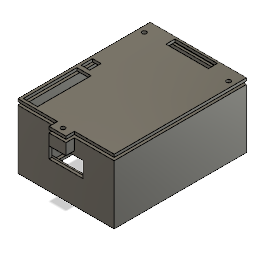
gpsAntenna v12 (Autodesk Fusion 360 design; units mm, degrees)
Autodesk Fusion 360 part; units mm, degrees
sketch "Sketch1" plane through (0, 0, 0) normal (0, 1, 0) x (1, 0, 0)
  line L0 (0, 0) -> (28.2, 0)
  line L1 (28.2, 0) -> (28.2, -28.2)
  line L2 (28.2, -28.2) -> (0, -28.2)
  line L3 (0, -28.2) -> (0, 0)
  line L4 (29.7, -29.7) -> (-1.5, -29.7)
  line L5 (-1.5, -29.7) -> (-1.5, 1.5)
  line L6 (-1.5, 1.5) -> (29.7, 1.5)
  line L7 (29.7, 1.5) -> (29.7, -29.7)
  line L8 (26.7, -1.5) -> (26.3464, -1.8536) construction
  line L9 (26.3464, -1.8536) -> (26.7, -2.2071) construction
  line L10 (26.7, -2.2071) -> (25.9929, -1.5)
  line L11 (26.7, -1.5) -> (27.0536, -1.1464) construction
  circle A0 centre (27.0536, -1.1464) radius 0.75
  line L12 (26.7, -26.7) -> (1.5, -1.5) construction
  line L13 (1.5, -26.7) -> (26.7, -1.5) construction
  circle A1 centre (1.1464, -1.1464) radius 0.75
  circle A2 centre (1.1464, -27.0536) radius 0.75
  circle A3 centre (27.0536, -27.0536) radius 0.75
  line L14 (27.2, -27.2) -> (1, -27.2)
  line L15 (1, -27.2) -> (1, -1)
  line L16 (1, -1) -> (27.2, -1)
  line L17 (27.2, -1) -> (27.2, -27.2)
  line L18 (27.2, -2.7071) -> (25.4929, -1)
  line L19 (2.7071, -1) -> (1, -2.7071)
  line L20 (1, -25.4929) -> (2.7071, -27.2)
  line L21 (25.4929, -27.2) -> (27.2, -25.4929)
  dimension "d1" = 28.2
  dimension "d2" = 28.2
  dimension "d5" = 1.5
  dimension "d12" = 1.5
  dimension "d15" = 1
  dimension "d17" = 360
  measures "d12" diameter of A0
extrude "Extrude1" add sketch "Sketch1" along normal blind 1 contours L0 L1 L2 L3 | L4 L5 L6 L7 | A3 L14 L17 L21 | A1 L15 L16 L19 | A2 L14 L15 L20 makes body 1
extrude "Extrude2" add sketch "Sketch1" along normal blind 5 contours L4 L5 L6 L7 bodies 1
extrude "Extrude3" add sketch "Sketch1" along normal blind 1 contours L10 A0 L16 L17 L18 bodies 1
extrude "Extrude4" add 1 faces at (-1, 5, 9.4) along direction (0, 1, 0) blind 1 on bodies 1 bodies 1
ref_plane "WorkPlane1" through (14.1, 6, 14.1) normal (0, 1, 0) x (0, 0, 1)
sketch "Sketch2" plane through (14.1, 6, 14.1) normal (0, 1, 0) x (1, 0, 0)
  line L0 (15.6, -15.6) -> (-15.6, -15.6)
  line L1 (15.6, -15.6) -> (15.6, -26) construction
  line L2 (15.6, -18.25) -> (-15.6, -18.25)
  line L3 (-15.6, -18.25) -> (-15.6, 18.25)
  line L4 (-15.6, 18.25) -> (15.6, 18.25)
  line L5 (15.6, 18.25) -> (15.6, -18.25)
  line L6 (15.6, -18.25) -> (-15.6, 18.25) construction
  line L7 (-15.6, -18.25) -> (15.6, 18.25) construction
  line L8 (16.1, -18.75) -> (-16.1, -18.75)
  line L9 (-16.1, -18.75) -> (-16.1, 18.75)
  line L10 (-16.1, 18.75) -> (16.1, 18.75)
  line L11 (16.1, 18.75) -> (16.1, -18.75)
  line L12 (17.1, -19.75) -> (-17.1, -19.75)
  line L13 (-17.1, -19.75) -> (-17.1, 19.75)
  line L14 (-17.1, 19.75) -> (17.1, 19.75)
  line L15 (17.1, 19.75) -> (17.1, -19.75)
  line L16 (-12.8, 25.4) -> (-12.8, -15.6)
  line L17 (-12.8, -15.6) -> (12.8, -15.6)
  line L18 (12.8, -15.6) -> (12.8, 25.4)
  line L19 (17.1, 19.75) -> (-17.1, 19.75)
  line L20 (-17.1, 19.75) -> (-17.1, 27.25)
  line L21 (-17.1, 27.25) -> (17.1, 27.25)
  line L22 (17.1, 27.25) -> (17.1, 19.75)
  line L23 (-12.8, 25.4) -> (12.8, 25.4)
  line L24 (12.8, 25.4) -> (12.8, 26.4)
  line L25 (12.8, 26.4) -> (-12.8, 26.4)
  line L26 (-12.8, 26.4) -> (-12.8, 25.4)
  dimension "d27" = 31.2
  dimension "d28" = 36.5
  dimension "d29" = 0.5
  dimension "d30" = 1.5
  dimension "d33" = 41
  dimension "d34" = 25.6
  dimension "d35" = 7.5
  dimension "d36" = 1
  measures "d29" distance of L2
  measures "d30" distance of L2
extrude "Extrude5" add sketch "Sketch2" against normal blind 6 separate body contours L8 L9 L10 L11 L12 L13 L14 L15 L16 L18 L19 | L14 L16 L18 L19 L20 L21 L22 L24 L25 L26 makes body 2
extrude "Extrude6" add 1 faces at (-1.5667, 6, -10.0333) along direction (0, 1, 0) blind 13 on bodies 2 bodies 2
extrude "Extrude7" add 1 faces at (-1.5, 2, 19.3) along direction (-1, 0, 0) blind 1.5 on bodies 1 bodies 1 2
extrude "Extrude8" add 1 faces at (29.7, 4, 19.3) along direction (1, 0, 0) blind 1.5 on bodies 1 bodies 1
ref_plane "WorkPlane2" through (14.1, 0, 10.35) normal (0, -1, 0) x (-1, 0, 0)
sketch "Sketch3" plane through (14.1, 0, 10.35) normal (0, -1, 0) x (1, 0, 0)
  line L0 (-17.1, -23.5) -> (17.1, -23.5)
  line L1 (17.1, -23.5) -> (17.1, 23.5)
  line L2 (17.1, 23.5) -> (-17.1, 23.5)
  line L3 (-17.1, 23.5) -> (-17.1, -23.5)
  line L4 (-12.8, -22.65) -> (12.8, -22.65)
  line L5 (12.8, -22.65) -> (12.8, -11.85)
  line L6 (12.8, -11.85) -> (-12.8, -11.85)
  line L7 (-12.8, -11.85) -> (-12.8, -22.65)
  line L8 (12.8, -22.65) -> (-12.8, -22.65)
  line L9 (0, -22.65) -> (0, -11.85)
  line L10 (-11.8, -21.65) -> (11.8, -21.65)
  line L11 (11.8, -21.65) -> (11.8, -12.85)
  line L12 (11.8, -12.85) -> (-11.8, -12.85)
  line L13 (-11.8, -12.85) -> (-11.8, -21.65)
  line L14 (-16.1, 19.35) -> (16.1, 19.35)
  line L15 (16.1, 19.35) -> (16.1, -11.85)
  line L16 (16.1, -11.85) -> (-16.1, -11.85)
  line L17 (-16.1, -11.85) -> (-16.1, 19.35)
  line L18 (-11.8, -12.85) -> (-7.8, -12.85)
  line L19 (-7.8, -12.85) -> (-7.8, -16.85)
  line L20 (-7.8, -16.85) -> (-11.8, -16.85)
  line L21 (-11.8, -16.85) -> (-11.8, -12.85)
  line L22 (0, -21.65) -> (11.8, -12.85) construction
  line L23 (5.9, -17.25) -> (5.9, -21.65) construction
  line L24 (5.9, -21.65) -> (5.9, -22.65) construction
  line L25 (5.9, -22.65) -> (5.9, -11.85)
  dimension "d46" = 1
  dimension "d53" = 4
  dimension "d54" = 4
  measures "d46" distance of L4
extrude "Extrude9" add sketch "Sketch3" against normal blind 0.5 contours L0 L1 L2 L3 | L4 L8 L9 L10 L25 | L4 L5 L6 L8 L10 L11 L12 L16 L25 | L9 L10 L12 L13 L19 L20 | L9 L10 L12 L25 | L6 L9 L12 L16 L25 | L10 L11 L12 L25 | L12 L13 L18 L19 L20 L21 bodies 1
extrude "Extrude10" add sketch "Sketch3" against normal blind 1 contours L9 L10 L12 L13 L19 L20 | L12 L13 L18 L19 L20 L21 bodies 1
extrude "Extrude11" add sketch "Sketch3" against normal blind 1 contours L4 L8 L9 L10 L25 | L4 L5 L6 L8 L10 L11 L12 L16 L25 | L9 L10 L12 L25 | L6 L9 L12 L16 L25 | L10 L11 L12 L25 bodies 1
extrude "Extrude12" add sketch "Sketch3" against normal blind 6 contours L12 L13 L18 L19 L20 L21 bodies 1
extrude "Extrude13" add 1 faces at (-1.2333, 19, -10.0333) along direction (0, 1, 0) blind 2 on bodies 1 bodies 1
ref_plane "WorkPlane3" through (14.1, 21, 10.35) normal (0, 1, 0) x (0, 0, 1)
sketch "Sketch4" plane through (14.1, 21, 10.35) normal (0, 1, 0) x (1, 0, 0)
  line L0 (17.1, -23.5) -> (-17.1, -23.5)
  line L1 (-17.1, -23.5) -> (-17.1, 23.5)
  line L2 (-17.1, 23.5) -> (17.1, 23.5)
  line L3 (17.1, 23.5) -> (17.1, -23.5)
  line L4 (-12.8, 15) -> (-17.1, 23.5)
  circle A0 centre (-14.95, 19.25) radius 0.75
  line L5 (16.1, 15) -> (16.1, -22.5)
  line L6 (0, 0) -> (0, -7)
  circle A1 centre (14.95, 19.25) radius 0.75
  line L7 (3, -26.5) -> (-3, -26.5)
  line L8 (-3, -26.5) -> (-3, -20.5)
  line L9 (-3, -20.5) -> (3, -20.5)
  line L10 (3, -20.5) -> (3, -26.5)
  line L11 (3, -26.5) -> (-3, -20.5) construction
  line L12 (-3, -26.5) -> (3, -20.5) construction
  line L13 (16.1, -22.5) -> (-16.1, -22.5) construction
  line L14 (0, -22.5) -> (0, -26.5) construction
  circle A2 centre (0, -24.5) radius 0.75
  line L15 (-17.1, -23.5) -> (-11.1, -23.5)
  line L16 (-11.1, -23.5) -> (-11.1, -8.5)
  line L17 (-11.1, -8.5) -> (-17.1, -8.5)
  line L18 (-17.1, -8.5) -> (-17.1, -23.5)
  line L19 (-16.1, -22.5) -> (-11.1, -22.5)
  line L20 (-11.1, -22.5) -> (-11.1, -8.5)
  line L21 (-11.1, -8.5) -> (-16.1, -8.5)
  line L22 (-16.1, -8.5) -> (-16.1, -22.5)
  line L23 (-7.5, 27.5) -> (7.5, 27.5)
  line L24 (7.5, 27.5) -> (7.5, 19.5)
  line L25 (7.5, 19.5) -> (-7.5, 19.5)
  line L26 (-7.5, 19.5) -> (-7.5, 27.5)
  line L27 (-7.5, 27.5) -> (7.5, 19.5) construction
  line L28 (7.5, 27.5) -> (-7.5, 19.5) construction
  line L29 (-21.1, 2) -> (-13.1, 2)
  line L30 (-13.1, 2) -> (-13.1, -2)
  line L31 (-13.1, -2) -> (-21.1, -2)
  line L32 (-21.1, -2) -> (-21.1, 2)
  line L33 (-21.1, 2) -> (-13.1, -2) construction
  line L34 (-13.1, 2) -> (-21.1, -2) construction
  line L35 (-16.1, 2) -> (-17.1, 2)
  line L36 (-17.1, 2) -> (-17.1, -2)
  line L37 (-17.1, -2) -> (-16.1, -2)
  line L38 (-16.1, -2) -> (-16.1, 2)
  line L39 (7.5, 22.65) -> (-7.5, 22.65)
  line L40 (-7.5, 22.65) -> (-7.5, 23.5)
  line L41 (-7.5, 23.5) -> (7.5, 23.5)
  line L42 (7.5, 23.5) -> (7.5, 22.65)
  dimension "d60" = 1.5
  dimension "d61" = 6
  dimension "d62" = 6
  dimension "d63" = 1.5
  dimension "d91" = 6
  dimension "d92" = 15
  dimension "d93" = 8
  dimension "d94" = 15
  dimension "d95" = 8
  dimension "d96" = 4
  measures "d60" diameter of A0
  measures "d63" diameter of A2
extrude "Extrude14" add sketch "Sketch4" against normal blind 4 contours L0 L7 L8 L10 | A2 bodies 1
extrude "Extrude15" cut sketch "Sketch4" against normal blind 3.5 contours A2 bodies 1
extrude "Extrude16" cut sketch "Sketch4" against normal blind 5 contours L4 A0 | L4 A0 | A1 bodies 1
extrude "Extrude17" add sketch "Sketch4" along normal blind 2 and the other way blind -1 separate body contours L0 L1 L2 L3 L8 L9 L10 L16 L17 L20 L21 L24 L25 L26 L29 L30 L31 L35 L37 L40 L42 | L0 L1 L15 L16 L17 L18 L19 L22 | L0 L8 L9 L10 | L0 L7 L8 L10 | L16 L17 L19 L20 L21 L22 | L1 L29 L31 L35 L36 L37 L38 | L29 L30 L31 L38 | L2 L24 L26 L39 L40 L41 L42 | L24 L25 L26 L39 makes body 3
extrude "Extrude18" add 1 faces at (4.9667, 6, -3.8333) along direction (0, 1, 0) blind 5 on bodies 1 bodies 1
extrude "Extrude19" cut sketch "Sketch3" against normal blind 1 contours L4 L8 L9 L10 L25 | L6 L9 L12 L16 L25 bodies 1
sketch "Sketch5" plane through (0, 0, -2.5) normal (0, 0, 1) x (1, 0, 0)
  line L0 (2.3, 0) -> (20, 0)
  line L1 (20, 0) -> (20, 1)
  line L2 (20, 1) -> (6.3, 1)
  line L3 (6.3, 1) -> (6.3, 11)
  line L4 (6.3, 11) -> (2.3, 11)
  line L5 (2.3, 11) -> (2.3, 0)
  line L6 (2.3, 11) -> (6.3, 11)
  line L7 (6.3, 11) -> (6.3, 9)
  line L8 (6.3, 9) -> (2.3, 9)
  line L9 (2.3, 9) -> (2.3, 11)
  line L10 (2.3, 9) -> (6.3, 9)
  line L11 (6.3, 9) -> (6.3, 5)
  line L12 (6.3, 5) -> (2.3, 5)
  line L13 (2.3, 5) -> (2.3, 9)
  dimension "d78" = 2
  dimension "d79" = 4
  dimension "d80" = 4
extrude "Extrude20" cut sketch "Sketch5" against normal blind 2.5 contours L3 L5 L8 L10 L11 L12 L13 bodies 1
ref_plane "WorkPlane4" through (14.1, 19, 36.85) normal (0, 0, 1) x (-1, 0, 0)
sketch "Sketch6" plane through (14.1, 19, 36.85) normal (0, 0, 1) x (1, 0, 0)
  line L0 (-3, -2) -> (3, -2)
  line L1 (3, -2) -> (3, 2)
  line L2 (3, 2) -> (-3, 2)
  line L3 (-3, 2) -> (-3, -2)
  line L4 (-3, -2) -> (-6, -2)
  line L5 (-6, -2) -> (6, -2)
  line L6 (-6, -2) -> (6, -2)
  line L7 (6, -2) -> (6, -2.5)
  line L8 (6, -2.5) -> (-6, -2.5)
  line L9 (-6, -2.5) -> (-6, -2)
  line L10 (-6, -2.5) -> (6, -2.5)
  line L11 (6, -2.5) -> (6, -7.5)
  line L12 (6, -7.5) -> (-6, -7.5)
  line L13 (-6, -7.5) -> (-6, -2.5)
  dimension "d84" = 3
  dimension "d99" = 12
  dimension "d100" = 0.5
  dimension "d101" = 5
  dimension "d102" = 12
extrude "Extrude22" cut sketch "Sketch4" along normal blind 5.438 contours L16 L17 L19 L20 L21 L22 | L29 L30 L31 L38 | L24 L25 L26 L39 bodies 3
extrude "Extrude23" cut sketch "Sketch6" against normal blind 4.467 contours L8 L10 L11 L12 L13 bodies 1
ref_plane "WorkPlane5" through (14.1, 6, 14.1) normal (0, 1, 0) x (0, 0, 1)
sketch "Sketch7" plane through (14.1, 6, 14.1) normal (0, 1, 0) x (1, 0, 0)
  line L0 (-14.1, 14.1) -> (14.1, 14.1)
  line L1 (14.1, 14.1) -> (14.1, -14.1)
  line L2 (14.1, -14.1) -> (-14.1, -14.1)
  line L3 (-14.1, -14.1) -> (-14.1, 14.1)
  line L4 (-16.1, 15.6) -> (16.1, 15.6)
  line L5 (16.1, 15.6) -> (16.1, -15.6)
  line L6 (16.1, -15.6) -> (-16.1, -15.6)
  line L7 (-16.1, -15.6) -> (-16.1, 15.6)
  line L8 (15.1, 15.1) -> (15.1, -15.1)
  line L9 (15.1, -15.1) -> (-15.1, -15.1)
  line L10 (-15.1, -15.1) -> (-15.1, 15.1)
  line L11 (-15.1, 15.1) -> (15.1, 15.1)
  dimension "d106" = 1
  measures "d106" distance of L1
extrude "Extrude24" cut sketch "Sketch7" against normal blind 5.5 contours L4 L5 L6 L7 bodies 1
sketch "Sketch8" plane through (0, 0, -4.65) normal (0, 0, 1) x (1, 0, 0)
  line L0 (26.9, 0.5) -> (30.2, 0.5)
  line L1 (30.2, 0.5) -> (30.2, 21)
  line L2 (30.2, 21) -> (26.9, 21)
  line L3 (26.9, 21) -> (26.9, 1)
  line L4 (26.9, 1) -> (26.9, 0.5)
  line L5 (30.2, 21) -> (-2, 21)
  line L6 (-2, 21) -> (-2, 0)
  line L7 (-2, 0) -> (30.2, 0)
  line L8 (30.2, 0) -> (30.2, 21)
  line L9 (14.1, 21) -> (14.1, 18)
  line L10 (26.9, 0.5) -> (30.2, 0.5)
  line L11 (30.2, 0.5) -> (30.2, 10.5)
  line L12 (30.2, 10.5) -> (26.9, 10.5)
  line L13 (26.9, 10.5) -> (26.9, 0.5)
  line L14 (-2, 10.5) -> (1.3, 10.5)
  line L15 (1.3, 10.5) -> (1.3, 0.5)
  line L16 (1.3, 0.5) -> (-2, 0.5)
  line L17 (-2, 0.5) -> (-2, 10.5)
extrude "Extrude25" cut sketch "Sketch8" against normal blind 7.65 contours L0 L1 L3 L4 L8 L10 L11 L12 L13 | L6 L14 L15 L16 L17 bodies 1
chamfer "Chamfer1" distance 7.5 angle 45 1 edges at (28.55, 10.5, -4.65) on bodies 1
chamfer "Chamfer2" distance 7.5 angle 45 1 edges at (-0.35, 10.5, -4.65) on bodies 1
extrude "Extrude26" cut 1 faces at (16.1, 11.5, 33.5167) along direction (0, -1, 0) blind 1.5 on bodies 1 bodies 1
extrude "Extrude27" add 1 faces at (16.1, 16.5, 33.5167) along direction (0, -1, 0) blind 1 on bodies 1 bodies 1
extrude "Extrude28" cut 1 faces at (1.3333, 22.3333, 18.85) along direction (0, 0, -1) blind 5 on bodies 3 bodies 3
ref_plane "WorkPlane6" through (14.1, 10.5, -13.15) normal (0, 0, -1) x (1, 0, 0)
sketch "Sketch9" plane through (14.1, 10.5, -13.15) normal (0, 0, -1) x (1, 0, 0)
  line L0 (17.1, -10.5) -> (-17.1, -10.5)
  line L1 (-17.1, -10.5) -> (-17.1, 10.5)
  line L2 (-17.1, 10.5) -> (17.1, 10.5)
  line L3 (17.1, 10.5) -> (17.1, -10.5)
  line L4 (17.1, -10.5) -> (12.8, -10.5)
  line L5 (12.8, -10.5) -> (12.8, 10.5)
  line L6 (12.8, 10.5) -> (17.1, 10.5)
  line L7 (17.1, 10.5) -> (17.1, -10.5)
  line L8 (-17.1, -10.5) -> (-12.8, -10.5)
  line L9 (-12.8, -10.5) -> (-12.8, 10.5)
  line L10 (-12.8, 10.5) -> (-17.1, 10.5)
  line L11 (-17.1, 10.5) -> (-17.1, -10.5)
  line L12 (12.8, -10.5) -> (10.8, -10.5)
  line L13 (10.8, -10.5) -> (10.8, -4.5)
  line L14 (10.8, -4.5) -> (12.8, -4.5)
  line L15 (12.8, -4.5) -> (12.8, -10.5)
  line L16 (12.8, -4.5) -> (10.8, -4.5)
  line L17 (10.8, -4.5) -> (10.8, -7.5)
  line L18 (10.8, -7.5) -> (12.8, -7.5)
  line L19 (12.8, -7.5) -> (12.8, -4.5)
  line L20 (6, 0.5) -> (-6, 0.5)
  line L21 (0, 0) -> (0, -3.5099)
  line L22 (-10.8, -7.5) -> (-12.8, -7.5)
  line L23 (-10.8, -10.5) -> (-10.8, -4.5)
  line L24 (-10.8, -4.5) -> (-12.8, -4.5)
  line L25 (-12.8, -10.5) -> (-12.8, 10.5)
  dimension "d120" = 4.3
  dimension "d121" = 4.3
  dimension "d122" = 6
  dimension "d123" = 2
  dimension "d124" = 3
extrude "Extrude29" add sketch "Sketch9" against normal blind 4.85 contours L5 L13 L14 L15 L16 L17 L18 L19 | L9 L22 L23 L24 L25 bodies 1
equation "d125 = -4 mm - 0.85 mm"
named bodies: "case", "lid"
